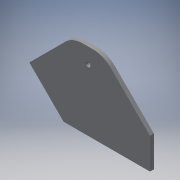
# Autodesk Inventor part: side Plate
Saved by Autodesk Inventor 2016 (Build 200138000, 138)
## iProperties
Created: 2016-11-04
Part Number: side Plate
Material: Generic
Document SubType Name: Modeling
Designer: william
Density: 1 g/cm^3
Appearance: Default
Author: william
Autodesk Inventor part; units mm, degrees
ref_plane "YZ Plane" through (0, 0, 0) normal (1, 0, 0) x (0, 1, 0)
ref_plane "XZ Plane" through (0, 0, 0) normal (0, 1, 0) x (-1, 0, 0)
ref_plane "XY Plane" through (0, 0, 0) normal (0, 0, 1) x (1, 0, 0)
sketch "Sketch1" plane through (0, 0, 0) normal (0, 1, 0) x (-1, 0, 0)
  line L0 (0, 0) -> (-140, 0)
  line L1 (-140, 0) -> (-140, 60)
  line L2 (-78.4315, 105) -> (-61.5685, 105)
  line L3 (0, 60) -> (-33.2843, 93.2843)
  line L4 (-140, 60) -> (-106.7157, 93.2843)
  arc A0 (-33.2843, 93.2843) -> (-61.5685, 105) centre (-61.5685, 65) ccw
  arc A1 (-78.4315, 105) -> (-106.7157, 93.2843) centre (-78.4315, 65) ccw
  circle A2 centre (-70, 90) radius 2.5
  line L5 (-85, 0) -> (-85, 5.2)
  line L6 (-85, 5.2) -> (-55, 5.2)
  line L7 (-55, 5.2) -> (-55, 0)
  circle A3 centre (-24, 30.7632) radius 11.5
  circle A4 centre (-39.5, 46.2632) radius 1.5
  circle A5 centre (-39.5, 15.2632) radius 1.5
  circle A6 centre (-8.5, 15.2632) radius 1.5
  circle A7 centre (-8.5, 46.2632) radius 1.5
  line L8 (-30, 0) -> (0, 0)
  line L9 (0, 0) -> (0, 5.2)
  line L10 (0, 5.2) -> (-30, 5.2)
  line L11 (-30, 5.2) -> (-30, 0)
  line L12 (-110, 0) -> (-140, 0)
  line L13 (-140, 0) -> (-140, 5.2)
  line L14 (-140, 5.2) -> (-110, 5.2)
  line L15 (-110, 5.2) -> (-110, 0)
  line L16 (0, 45) -> (5.2, 45)
  line L17 (5.2, 45) -> (5.2, 15)
  line L18 (5.2, 15) -> (0, 15)
  line L19 (0, 60) -> (0, 45)
  line L20 (0, 15) -> (0, 0)
  point P0 (-45, 105)
  point P1 (-95, 105)
  point P2 (-70, 105)
  dimension "d0" = 140
  dimension "d1" = 60
  dimension "d3" = 135
  dimension "d4" = 50
  dimension "d5" = 40
  dimension "d8" = 5
  dimension "d12" = 90
  dimension "d13" = 30
  dimension "d14" = 15
  dimension "d15" = 5.2
  dimension "d16" = 23
  dimension "d17" = 75
  dimension "d18" = 3
  dimension "d19" = 15.5
  dimension "d20" = 15.5
  dimension "d23" = 360
  dimension "d25" = 30
  dimension "d26" = 5.2
  dimension "d28" = 30
  dimension "d29" = 5.2
  dimension "d35" = 30
  dimension "d36" = 15
  dimension "d37" = 24
  dimension "d38" = 15
  dimension "d39" = 5.2
  dimension "d40" = 5.2
  dimension "d41" = 70
  constraints: 42 end point, 10 point on line, 8 centre point, 8 parallel, 6 perpendicular, 4 horizontal, 4 point on circle, 4 tangent, 1 equal radius, 1 midpoint, 1 vertical, 1 vertical alignment, 9 other
  measures "d0" distance of L0.start L0.end
  measures "d1" distance of L0.end L1.end
  measures "d3" angle of L1 L4
  measures "d4" distance of point (-95, 105) point (-45, 105)
  measures "d5" radius of A0
  measures "d8" diameter of A2
  measures "d12" distance from line of A2.centre L0
  measures "d13" distance of L5.end L6.end
  measures "d14" distance from line of point (-70, 105) L5
  measures "d15" distance between parallel lines of L0 L6
  measures "d16" diameter of A3
  measures "d17" distance of A3.centre A2.centre
  measures "d18" diameter of A4
  measures "d19" horizontal distance of A3.centre A4.centre
  measures "d20" horizontal distance of A3.centre A4.centre
  measures "d25" distance of L9.end L10.end
  measures "d26" distance between parallel lines of L0 L10
  measures "d28" distance of L13.end L14.end
  measures "d29" distance of L14.end L12.start
  measures "d35" distance between parallel lines of L18 L16
  measures "d36" distance between parallel lines of L0 L18
  measures "d37" distance from line of L20 A3.centre
  measures "d38" distance of L3.start L16.start
  measures "d39" distance of L17.end L18.end
  measures "d40" distance of L16.start L16.end
  measures "d41" distance from line of L1 A2.centre
extrude "Extrusion3" add sketch "Sketch1" along normal blind 5.2 contours L0 L7 L6 L5 L15 L14 L1 L4 A1 L2 A0 L3 L19 L16 L17 L18 L20 L10 L11
body "Solid2"
